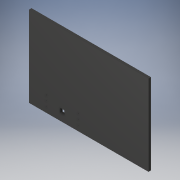
# Autodesk Inventor part: BA12
Saved by Autodesk Inventor 2017 (Build 210142000, 142)
## iProperties
Created: 2018-10-18
Part Number: BA12
Material: ABS Plastic
Document SubType Name: Modeling
Designer: Dell
Density: 1.06 g/cm^3
Appearance: Smooth - Black
Author: Dell
Autodesk Inventor part; units mm, degrees
ref_plane "YZ Plane" through (0, 0, 0) normal (1, 0, 0) x (0, 1, 0)
ref_plane "XZ Plane" through (0, 0, 0) normal (0, 1, 0) x (-1, 0, 0)
ref_plane "XY Plane" through (0, 0, 0) normal (0, 0, 1) x (1, 0, 0)
sketch "Sketch1" plane through (0, 0, 0) normal (0, 0, 1) x (1, 0, 0)
  line L0 (0, 0) -> (525.78, 0)
  line L1 (525.78, 0) -> (525.78, 355.6)
  line L2 (525.78, 355.6) -> (0, 355.6)
  line L3 (0, 355.6) -> (0, 0)
  dimension "d0" = 525.78
  dimension "d1" = 355.6
  constraints: 8 end point, 2 parallel, 1 horizontal, 1 perpendicular
  measures "d0" distance of L2.end L1.end
  measures "d1" distance of L1.end L0.end
extrude "Extrusion1" add sketch "Sketch1" along normal blind 10
sketch "Sketch9" plane through (0, 0, 10) normal (0, 0, 1) x (1, 0, 0)
  line L0 (525.78, 0) -> (525.78, 355.6) construction
  line L1 (0, 0) -> (525.78, 0) construction
  line L2 (525.78, 0) -> (525.78, 88.9)
  line L3 (525.78, 88.9) -> (0, 88.9) construction
  line L4 (0, 88.9) -> (0, 0) construction
  line L5 (76.2, 21.95) -> (76.2, 66.95) construction
  line L6 (76.2, 66.95) -> (216.2, 66.95) construction
  line L7 (216.2, 66.95) -> (216.2, 21.95) construction
  line L8 (216.2, 21.95) -> (76.2, 21.95) construction
  circle A0 centre (76.2, 66.95) radius 2.3812
  circle A1 centre (76.2, 44.45) radius 2.3812
  circle A2 centre (76.2, 21.95) radius 2.3812
  circle A3 centre (216.2, 21.95) radius 2.3813
  circle A4 centre (216.2, 44.45) radius 2.3813
  circle A5 centre (216.2, 66.95) radius 2.3813
  line L9 (76.2, 44.45) -> (216.2, 44.45) construction
  line L10 (146.2, 66.95) -> (146.2, 21.95) construction
  line L11 (136.2, 49.45) -> (136.2, 29.45)
  line L12 (136.2, 29.45) -> (156.2, 29.45)
  line L13 (156.2, 29.45) -> (156.2, 49.45)
  line L14 (156.2, 49.45) -> (136.2, 49.45)
  point P0 (0, 44.45)
  dimension "d41" = 45
  dimension "d42" = 140
  dimension "d43" = 4.7625
  dimension "d44" = 4.7625
  dimension "d45" = 4.7625
  dimension "d46" = 4.7625
  dimension "d47" = 4.7625
  dimension "d48" = 4.7625
  dimension "d49" = 60
  dimension "d50" = 7.5
  dimension "d51" = 20
  dimension "d52" = 20
  dimension "d53" = 76.2
  dimension "d54" = 88.9
  constraints: 28 end point, 6 centre point, 6 parallel, 5 midpoint, 4 coincident, 3 perpendicular, 1 horizontal, 1 horizontal alignment, 1 point on line
  measures "d41" distance of L6.end L8.start
  measures "d42" distance of L5.end L6.end
  measures "d43" diameter of A0
  measures "d44" diameter of A1
  measures "d45" diameter of A2
  measures "d46" diameter of A3
  measures "d47" diameter of A4
  measures "d48" diameter of A5
  measures "d49" distance from line of L9.end L13
  measures "d50" distance between parallel lines of L8 L12
  measures "d51" distance of L14.start L11.start
  measures "d52" distance of L11.start L11.end
  measures "d53" distance between parallel lines of L4 L5
  measures "d54" distance of L3.end L1.start
extrude "Extrusion8" cut sketch "Sketch9" against normal through all
body "Solid1"
